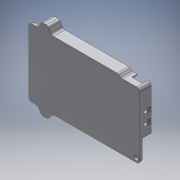
# Autodesk Inventor part: Case_superior_nuevo
Saved by Autodesk Inventor 2019 (Build 230136000, 136)
## iProperties
Created: 2018-11-21
Part Number: Case_superior_nuevo
Material: Steel, Mild, Welded
Document SubType Name: Modeling
Designer: cadcae
Density: 7.85 g/cm^3
Appearance: Smooth - White
Author: cadcae
Autodesk Inventor part; units mm, degrees
ref_plane "YZ Plane" through (0, 0, 0) normal (1, 0, 0) x (0, 1, 0)
ref_plane "XZ Plane" through (0, 0, 0) normal (0, 1, 0) x (-1, 0, 0)
ref_plane "XY Plane" through (0, 0, 0) normal (0, 0, 1) x (1, 0, 0)
sketch "Sketch1" plane through (0, 0, 0) normal (0, 0, 1) x (1, 0, 0)
  line L0 (26.8957, -31.2712) -> (26.8957, -23.2912) projected
  line L1 (26.8957, -23.2912) -> (21.7957, -23.2912) projected
  arc A0 (21.7957, -23.2912) -> (19.7957, -25.2912) centre (21.7957, -25.2912) ccw projected
  line L2 (19.7957, -25.2912) -> (19.7957, -28.2712) projected
  line L3 (19.7957, -28.2712) -> (1.7957, -28.2712) projected
  line L4 (1.7957, -28.2712) -> (1.7957, -25.2912) projected
  arc A1 (1.7957, -25.2912) -> (-0.2043, -23.2912) centre (-0.2043, -25.2912) ccw projected
  line L5 (-0.2043, -23.2912) -> (-1.3443, -23.2912) projected
  arc A2 (-1.3443, -23.2912) -> (-3.3443, -25.2912) centre (-1.3443, -25.2912) ccw projected
  line L6 (-3.3443, -25.2912) -> (-3.3443, -29.2712) projected
  line L7 (-3.3443, -29.2712) -> (-48.3643, -29.2712) projected
  line L8 (-48.3643, -29.2712) -> (-48.3643, -13.3852) projected
  line L9 (-48.3643, -13.3852) -> (-51.3643, -13.3852) projected
  line L10 (-51.3643, -13.3852) -> (-51.3643, -28.2712) projected
  arc A3 (-51.3643, -28.2712) -> (-48.3643, -31.2712) centre (-48.3643, -28.2712) ccw projected
  line L11 (-48.3643, -31.2712) -> (-44.5605, -31.2712) projected
  arc A4 (-41.9624, -32.7712) -> (-44.5605, -31.2712) centre (-44.5605, -34.2712) ccw projected
  line L12 (-40.2304, -35.7712) -> (-41.9624, -32.7712) projected
  arc A5 (-40.2304, -35.7712) -> (-37.6323, -37.2712) centre (-37.6323, -34.2712) ccw projected
  line L13 (-35.0964, -37.2712) -> (-37.6323, -37.2712) projected
  arc A6 (-35.0964, -37.2712) -> (-32.4983, -35.7712) centre (-35.0964, -34.2712) ccw projected
  line L14 (-30.7663, -32.7712) -> (-32.4983, -35.7712) projected
  arc A7 (-28.1682, -31.2712) -> (-30.7663, -32.7712) centre (-28.1682, -34.2712) ccw projected
  line L15 (-28.1682, -31.2712) -> (26.8957, -31.2712) projected
  line L16 (-45.3643, 31.7788) -> (-45.3643, 28.7788) projected
  line L17 (-45.3643, 28.7788) -> (22.8137, 28.7788) projected
  line L18 (22.8137, 28.7788) -> (24.1137, 30.2788) projected
  line L19 (24.1137, 30.2788) -> (28.1137, 30.2788) projected
  line L20 (28.1137, 30.2788) -> (29.4137, 28.7788) projected
  line L21 (29.4137, 28.7788) -> (39.3157, 28.7788) projected
  line L22 (39.3157, 28.7788) -> (39.3157, 29.7218) projected
  line L23 (39.3157, 29.7218) -> (35.9475, 29.7218) projected
  arc A8 (34.4475, 30.1238) -> (35.9475, 29.7218) centre (35.9475, 32.7218) ccw projected
  line L24 (34.4475, 30.1238) -> (32.277, 31.3769) projected
  arc A9 (32.277, 31.3769) -> (30.777, 31.7788) centre (30.777, 28.7788) ccw projected
  line L25 (30.777, 31.7788) -> (-28.1682, 31.7788) projected
  arc A10 (-30.7663, 33.2788) -> (-28.1682, 31.7788) centre (-28.1682, 34.7788) ccw projected
  line L26 (-32.4983, 36.2788) -> (-30.7663, 33.2788) projected
  arc A11 (-32.4983, 36.2788) -> (-35.0964, 37.7788) centre (-35.0964, 34.7788) ccw projected
  line L27 (-37.6323, 37.7788) -> (-35.0964, 37.7788) projected
  arc A12 (-37.6323, 37.7788) -> (-40.2304, 36.2788) centre (-37.6323, 34.7788) ccw projected
  line L28 (-41.9624, 33.2788) -> (-40.2304, 36.2788) projected
  arc A13 (-44.5605, 31.7788) -> (-41.9624, 33.2788) centre (-44.5605, 34.7788) ccw projected
  line L29 (-44.5605, 31.7788) -> (-45.3643, 31.7788) projected
  line L30 (48.8957, -11.2712) -> (51.8957, -11.2712) projected
  line L31 (51.8957, -11.2712) -> (51.8957, 26.7218) projected
  arc A14 (51.8957, 26.7218) -> (48.8957, 29.7218) centre (48.8957, 26.7218) ccw projected
  line L32 (48.8957, 29.7218) -> (48.3157, 29.7218) projected
  line L33 (48.3157, 29.7218) -> (48.3157, 28.7788) projected
  line L34 (48.3157, 28.7788) -> (48.8957, 28.7788) projected
  line L35 (48.8957, 28.7788) -> (48.8957, -11.2712) projected
  line L36 (-48.3643, 6.9348) -> (-51.3643, 6.9348) projected
  line L37 (-51.3643, 6.9348) -> (-51.3643, -4.2412) projected
  line L38 (-51.3643, -4.2412) -> (-48.3643, -4.2412) projected
  line L39 (-48.3643, -4.2412) -> (-48.3643, 6.9348) projected
  line L40 (-48.3643, -13.3852) -> (-51.3643, -13.3852)
  line L41 (-51.3643, -4.2412) -> (-48.3643, -4.2412)
  line L42 (-48.3643, 6.9348) -> (-51.3643, 6.9348)
  line L43 (-51.3643, 6.9348) -> (-51.3643, 16.0788)
  line L44 (-51.3643, 16.0788) -> (-48.3643, 16.0788)
  line L45 (-48.3643, 16.0788) -> (-48.3643, 6.9348)
  line L46 (-48.3643, 18.7788) -> (-51.3643, 18.7788) projected
  line L47 (-51.3643, 18.7788) -> (-51.3643, 16.0788) projected
  line L48 (-51.3643, 16.0788) -> (-48.3643, 16.0788) projected
  line L49 (-48.3643, 16.0788) -> (-48.3643, 18.7788) projected
  line L50 (-48.3643, -13.3852) -> (-51.3643, -13.3852)
  line L51 (-51.3643, -13.3852) -> (-51.3643, -4.2412)
  line L52 (-51.3643, -4.2412) -> (-48.3643, -4.2412)
  line L53 (-48.3643, -4.2412) -> (-48.3643, -13.3852)
  line L54 (48.3157, 29.7218) -> (48.3157, 28.7788) projected
  line L55 (39.3157, 29.7218) -> (48.3157, 29.7218) projected
  line L56 (39.3157, 28.7788) -> (39.3157, 29.7218) projected
  line L57 (48.3157, 28.7788) -> (39.3157, 28.7788) projected
  point P0 (0, 0)
  constraints: 20 end point, 6 point on line, 5 parallel, 3 horizontal, 2 perpendicular
extrude "Extrusion1" add sketch "Sketch1" along normal blind 8.6
sketch "Sketch2" plane through (0, 0, 8.6) normal (0, 0, 1) x (1, 0, 0)
  line L0 (26.8957, -31.2712) -> (26.8957, -23.2912) projected
  line L1 (26.8957, -23.2912) -> (21.7957, -23.2912) projected
  arc A0 (21.7957, -23.2912) -> (19.7957, -25.2912) centre (21.7957, -25.2912) ccw projected
  line L2 (19.7957, -25.2912) -> (19.7957, -28.2712) projected
  line L3 (19.7957, -28.2712) -> (1.7957, -28.2712) projected
  line L4 (1.7957, -28.2712) -> (1.7957, -25.2912) projected
  arc A1 (1.7957, -25.2912) -> (-0.2043, -23.2912) centre (-0.2043, -25.2912) ccw projected
  line L5 (-0.2043, -23.2912) -> (-1.3443, -23.2912) projected
  arc A2 (-1.3443, -23.2912) -> (-3.3443, -25.2912) centre (-1.3443, -25.2912) ccw projected
  line L6 (-3.3443, -25.2912) -> (-3.3443, -29.2712) projected
  line L7 (-3.3443, -29.2712) -> (-48.3643, -29.2712) projected
  line L8 (-48.3643, -29.2712) -> (-48.3643, 18.7788) projected
  line L9 (-51.3643, 18.7788) -> (-51.3643, -28.2712) projected
  arc A3 (-51.3643, -28.2712) -> (-48.3643, -31.2712) centre (-48.3643, -28.2712) ccw projected
  line L10 (-48.3643, -31.2712) -> (-44.5605, -31.2712) projected
  arc A4 (-41.9624, -32.7712) -> (-44.5605, -31.2712) centre (-44.5605, -34.2712) ccw projected
  line L11 (-41.9624, -32.7712) -> (-40.2304, -35.7712) projected
  arc A5 (-40.2304, -35.7712) -> (-37.6323, -37.2712) centre (-37.6323, -34.2712) ccw projected
  line L12 (-37.6323, -37.2712) -> (-35.0964, -37.2712) projected
  arc A6 (-35.0964, -37.2712) -> (-32.4983, -35.7712) centre (-35.0964, -34.2712) ccw projected
  line L13 (-32.4983, -35.7712) -> (-30.7663, -32.7712) projected
  arc A7 (-28.1682, -31.2712) -> (-30.7663, -32.7712) centre (-28.1682, -34.2712) ccw projected
  line L14 (-28.1682, -31.2712) -> (26.8957, -31.2712) projected
  line L15 (-48.3643, 18.7788) -> (-51.3643, 18.7788) projected
  line L16 (-48.3643, 28.7788) -> (-45.3643, 28.7788) projected
  line L17 (-45.3643, 28.7788) -> (-45.3643, 31.7788) projected
  line L18 (-45.3643, 31.7788) -> (-48.3643, 31.7788) projected
  arc A8 (-48.3643, 31.7788) -> (-51.3643, 28.7788) centre (-48.3643, 28.7788) ccw projected
  line L19 (-51.3643, 28.7788) -> (-51.3643, 18.7788) projected
  line L20 (-51.3643, 18.7788) -> (-48.3643, 18.7788) projected
  line L21 (-48.3643, 18.7788) -> (-48.3643, 28.7788) projected
  line L22 (29.4137, 28.7788) -> (48.8957, 28.7788) projected
  line L23 (48.8957, 28.7788) -> (48.8957, -11.2712) projected
  line L24 (48.8957, -11.2712) -> (51.8957, -11.2712) projected
  line L25 (51.8957, -11.2712) -> (51.8957, 26.7218) projected
  arc A9 (51.8957, 26.7218) -> (48.8957, 29.7218) centre (48.8957, 26.7218) ccw projected
  line L26 (48.8957, 29.7218) -> (35.9475, 29.7218) projected
  arc A10 (34.4475, 30.1238) -> (35.9475, 29.7218) centre (35.9475, 32.7218) ccw projected
  line L27 (34.4475, 30.1238) -> (32.277, 31.3769) projected
  arc A11 (32.277, 31.3769) -> (30.777, 31.7788) centre (30.777, 28.7788) ccw projected
  line L28 (30.777, 31.7788) -> (-28.1682, 31.7788) projected
  arc A12 (-30.7663, 33.2788) -> (-28.1682, 31.7788) centre (-28.1682, 34.7788) ccw projected
  line L29 (-30.7663, 33.2788) -> (-32.4983, 36.2788) projected
  arc A13 (-32.4983, 36.2788) -> (-35.0964, 37.7788) centre (-35.0964, 34.7788) ccw projected
  line L30 (-35.0964, 37.7788) -> (-37.6323, 37.7788) projected
  arc A14 (-37.6323, 37.7788) -> (-40.2304, 36.2788) centre (-37.6323, 34.7788) ccw projected
  line L31 (-40.2304, 36.2788) -> (-41.9624, 33.2788) projected
  arc A15 (-44.5605, 31.7788) -> (-41.9624, 33.2788) centre (-44.5605, 34.7788) ccw projected
  line L32 (-44.5605, 31.7788) -> (-45.3643, 31.7788) projected
  line L33 (-45.3643, 31.7788) -> (-45.3643, 28.7788) projected
  line L34 (-45.3643, 28.7788) -> (22.8137, 28.7788) projected
  line L35 (22.8137, 28.7788) -> (24.1137, 30.2788) projected
  line L36 (24.1137, 30.2788) -> (28.1137, 30.2788) projected
  line L37 (28.1137, 30.2788) -> (29.4137, 28.7788) projected
  arc A16 (48.8957, -31.2712) -> (51.8957, -28.2712) centre (48.8957, -28.2712) ccw projected
  line L38 (51.8957, -28.2712) -> (51.8957, -11.2712) projected
  line L39 (51.8957, -11.2712) -> (48.8957, -11.2712) projected
  line L40 (48.8957, -11.2712) -> (48.8957, -23.2912) projected
  line L41 (48.8957, -23.2912) -> (26.8957, -23.2912) projected
  line L42 (26.8957, -23.2912) -> (26.8957, -31.2712) projected
  line L43 (26.8957, -31.2712) -> (48.8957, -31.2712) projected
  point P0 (0, 0)
extrude "Extrusion2" add sketch "Sketch2" along normal blind 2 contours L14 A7 L13 A6 L12 A5 L11 A4 L10 A3 L9 L15 L8 L7 L6 A2 L5 A1 L4 L3 L2 A0 L1 L0 | L0 L41 L40 L24 L38 A16 L43 | L23 L22 L37 L36 L35 L34 L17 L32 A15 L31 A14 L30 A13 L29 A12 L28 A11 L27 A10 L26 A9 L25 L24 | L16 L21 L15 L19 A8 L18 L17
sketch "Sketch3" plane through (-48.3643, -29.2712, 0) normal (1, 0, 0) x (0, 0, -1)
  line L0 (0, 48.05) -> (0, 1) projected
  line L1 (0, 1) -> (-10.6, 1) projected
  line L2 (-10.6, 58.05) -> (-10.6, 1) projected
  line L3 (-8.6, 58.05) -> (-10.6, 58.05) projected
  line L4 (-8.6, 58.05) -> (-8.6, 48.05) projected
  line L5 (0, 48.05) -> (-8.6, 48.05) projected
  line L6 (-8.6, 61.05) -> (-8.6, 58.05) projected
  line L7 (-8.6, 58.05) -> (-10.6, 58.05) projected
  line L8 (-10.6, 61.05) -> (-10.6, 58.05) projected
  line L9 (-8.6, 61.05) -> (-10.6, 61.05) projected
  line L10 (0, 1) -> (0, -2) projected
  line L11 (0, -2) -> (-10.6, -2) projected
  line L12 (-10.6, 1) -> (-10.6, -2) projected
  line L13 (0, 1) -> (-10.6, 1) projected
  line L14 (-10.6, -2) -> (-8.6, -2)
  line L15 (-8.6, -2) -> (-8.6, 61.05)
  line L16 (-8.6, 61.05) -> (-10.6, 61.05)
  line L17 (-10.6, 61.05) -> (-10.6, -2)
  point P0 (0, 29.2712)
  dimension "d4" = 2
  constraints: 8 end point, 2 parallel, 1 horizontal, 1 perpendicular
  measures "d4" distance of L15.end L8.start
extrude "Extrusion3" add sketch "Sketch3" along normal up to surface (97.26 mm away) contours L15 L1 L2 L3 L4 | L15 L11 L12 L1
extrude "Extrusion4" add sketch "Sketch3" along normal up to surface (77.778 mm away) contours L3 L8 L9 L6
sketch "Sketch4" plane through (-51.3643, -28.2712, 0) normal (-1, 0, 0) x (0, 0, 1)
  circle A0 centre (0, 39.778) radius 4.572
  circle A1 centre (0, 19.458) radius 4.572
  line L0 (0, 47.05) -> (0, 0) projected
  line L1 (0, 0) -> (10.6, 0) projected
  line L2 (10.6, 57.05) -> (10.6, 0) projected
  line L3 (8.6, 57.05) -> (10.6, 57.05) projected
  line L4 (8.6, 57.05) -> (8.6, 47.05) projected
  line L5 (0, 47.05) -> (8.6, 47.05) projected
  line L6 (0, 47.05) -> (0, 0) projected
  point P0 (0, 28.2712)
  dimension "d9" = 7.272
  dimension "d10" = 20.32
  dimension "d13" = 9.144
  constraints: 2 centre point, 1 equal radius, 1 point on line, 1 vertical alignment
  measures "d9" distance from line of A0.centre L5
  measures "d10" distance of A1.centre A0.centre
  measures "d13" diameter of A0
extrude "Extrusion5" cut sketch "Sketch4" against normal blind 10 contours A0 L0 | L0 A0 | L0 A1 | A1 L0
sketch "Sketch5" plane through (35.9475, 29.7218, 0) normal (0, 1, 0) x (1, 0, 0)
  line L0 (12.3682, -4.5974) -> (3.3682, -4.5974)
  line L1 (3.3682, -4.5974) -> (3.3682, 0)
  line L2 (3.3682, 0) -> (12.3682, 0)
  line L3 (12.3682, 0) -> (12.3682, -4.5974)
  line L4 (12.9482, 0) -> (0, 0) projected
  line L5 (0, 0) -> (0, -10.6) projected
  line L6 (12.9482, -10.6) -> (0, -10.6) projected
  line L7 (12.9482, 0) -> (12.9482, -10.6) projected
  line L8 (15.9482, 0) -> (12.9482, 0) projected
  line L9 (12.9482, 0) -> (12.9482, -10.6) projected
  line L10 (15.9482, -10.6) -> (12.9482, -10.6) projected
  line L11 (15.9482, 0) -> (15.9482, -10.6) projected
  line L12 (12.9482, 0) -> (0, 0) projected
  point P0 (-35.9475, 0)
  dimension "d14" = 4.5974
  dimension "d15" = 3.58
  dimension "d16" = 9
  constraints: 8 end point, 2 parallel, 1 horizontal, 1 perpendicular, 1 point on line
  measures "d14" distance between parallel lines of L4 L0
  measures "d15" distance between parallel lines of L3 L11
  measures "d16" distance of L1.end L2.end
extrude "Extrusion6" cut sketch "Sketch5" against normal up to next contours L0 L1 L2 L3
sketch "Sketch6" plane through (51.8957, -11.2712, 0) normal (1, 0, 0) x (0, 0, -1)
  line L0 (0, 0) -> (0, 37.993) projected
  line L1 (0, 37.993) -> (-10.6, 37.993) projected
  line L2 (-10.6, -17) -> (-10.6, 37.993) projected
  line L3 (-8.6, -17) -> (-10.6, -17) projected
  line L4 (-8.6, -17) -> (-8.6, 0) projected
  line L5 (0, 0) -> (-8.6, 0) projected
  circle A0 centre (-5.3, 10) radius 1.5
  circle A1 centre (-5.3, 20) radius 1.5
  point P0 (0, 11.2712)
  point P1 (-5.3, 37.993)
  dimension "d19" = 10
  dimension "d20" = 10
  dimension "d21" = 3
  constraints: 2 centre point, 2 vertical alignment, 1 equal radius, 1 midpoint
  measures "d19" distance from line of L5 A0.centre
  measures "d20" distance of A1.centre A0.centre
  measures "d21" diameter of A0
extrude "Extrusion7" cut sketch "Sketch6" against normal up to next contours A0 | A1
sketch "Sketch7" plane through (51.8957, -11.2712, 0) normal (1, 0, 0) x (0, 0, -1)
  line L0 (-3.2, 7.3511) -> (-3.2, 12.6489) construction
  line L1 (-3.2, 12.6489) -> (-0.5947, 12.6489) construction
  line L2 (-0.5947, 12.6489) -> (-0.5947, 7.3511) construction
  line L3 (-0.5947, 7.3511) -> (-3.2, 7.3511) construction
  line L4 (-3.2, 17.6246) -> (-3.2, 22.3754) construction
  line L5 (-3.2, 22.3754) -> (-0.5987, 22.3754) construction
  line L6 (-0.5987, 22.3754) -> (-0.5987, 17.6246) construction
  line L7 (-0.5987, 17.6246) -> (-3.2, 17.6246) construction
  circle A0 centre (-5.3, 10) radius 1.5 projected
  circle A1 centre (-5.3, 20) radius 1.5 projected
  line L8 (0, 0) -> (0, 37.993) projected
  line L9 (0, 37.993) -> (-10.6, 37.993) projected
  line L10 (-10.6, -17) -> (-10.6, 37.993) projected
  line L11 (-8.6, -17) -> (-10.6, -17) projected
  line L12 (-8.6, -17) -> (-8.6, 0) projected
  line L13 (0, 0) -> (-8.6, 0) projected
  spline S0 degree 2 poles (-1.8973, 9.8855) (-1.2895, 9.8855) (-0.5947, 9.2372) (-0.5947, 8.674) knots 0 0 0 1 2 2 2
  spline S1 degree 2 poles (-0.5947, 8.674) (-0.5947, 8.1088) (-1.2977, 7.4645) (-1.8973, 7.4645) knots 0 0 0 1 2 2 2
  spline S2 degree 2 poles (-1.8973, 7.4645) (-2.499, 7.4645) (-3.2, 8.1088) (-3.2, 8.674) knots 0 0 0 1 2 2 2
  spline S3 degree 2 poles (-3.2, 8.674) (-3.2, 9.2372) (-2.5031, 9.8855) (-1.8973, 9.8855) knots 0 0 0 1 2 2 2
  spline S4 degree 2 poles (-1.8973, 9.2372) (-2.1222, 9.2372) (-2.4362, 9.1461) (-2.5355, 9.0671) knots 0 0 0 1 2 2 2
  spline S5 degree 2 poles (-2.5355, 9.0671) (-2.6388, 8.988) (-2.728, 8.7855) (-2.728, 8.6761) knots 0 0 0 1 2 2 2
  spline S6 degree 2 poles (-2.728, 8.6761) (-2.728, 8.5606) (-2.6449, 8.3722) (-2.5395, 8.285) knots 0 0 0 1 2 2 2
  spline S7 degree 2 poles (-2.5395, 8.285) (-2.4423, 8.2081) (-2.1202, 8.1128) (-1.8973, 8.1128) knots 0 0 0 1 2 2 2
  spline S8 degree 2 poles (-1.8973, 8.1128) (-1.6664, 8.1128) (-1.3625, 8.204) (-1.2592, 8.283) knots 0 0 0 1 2 2 2
  spline S9 degree 2 poles (-1.2592, 8.283) (-1.1558, 8.362) (-1.0667, 8.5667) (-1.0667, 8.6761) knots 0 0 0 1 2 2 2
  spline S10 degree 2 poles (-1.0667, 8.6761) (-1.0667, 8.7875) (-1.1619, 8.9941) (-1.2632, 9.0691) knots 0 0 0 1 2 2 2
  spline S11 degree 2 poles (-1.2632, 9.0691) (-1.3726, 9.1501) (-1.6623, 9.2372) (-1.8973, 9.2372) knots 0 0 0 1 2 2 2
  line L14 (-0.6473, 12.3997) -> (-0.6473, 11.796)
  line L15 (-0.6473, 11.796) -> (-2.3896, 10.8316)
  line L16 (-2.3896, 10.8316) -> (-0.6473, 10.8316)
  line L17 (-0.6473, 10.8316) -> (-0.6473, 10.2583)
  line L18 (-0.6473, 10.2583) -> (-3.1473, 10.2583)
  line L19 (-3.1473, 10.2583) -> (-3.1473, 11.0282)
  line L20 (-3.1473, 11.0282) -> (-1.715, 11.8264)
  line L21 (-1.715, 11.8264) -> (-3.1473, 11.8264)
  line L22 (-3.1473, 11.8264) -> (-3.1473, 12.3997)
  line L23 (-3.1473, 12.3997) -> (-0.6473, 12.3997)
  line L24 (-0.6514, 19.7154) -> (-0.6514, 17.8778)
  line L25 (-0.6514, 17.8778) -> (-1.0586, 17.8778)
  spline S12 degree 2 poles (-1.0586, 17.8778) (-1.245, 18.1108) (-1.5732, 18.4836) (-1.7211, 18.6234) knots 0 0 0 1 2 2 2
  spline S13 degree 2 poles (-1.7211, 18.6234) (-1.9135, 18.8077) (-2.2073, 18.9718) (-2.3613, 18.9718) knots 0 0 0 1 2 2 2
  spline S14 degree 2 poles (-2.3613, 18.9718) (-2.5355, 18.9718) (-2.7219, 18.7632) (-2.7219, 18.5768) knots 0 0 0 1 2 2 2
  spline S15 degree 2 poles (-2.7219, 18.5768) (-2.7219, 18.4816) (-2.6753, 18.3114) (-2.6388, 18.2243) knots 0 0 0 1 2 2 2
  spline S16 degree 2 poles (-2.6388, 18.2243) (-2.6003, 18.1392) (-2.5193, 18.0176) (-2.499, 17.9872) knots 0 0 0 1 2 2 2
  line L26 (-2.499, 17.9872) -> (-2.499, 17.9386)
  line L27 (-2.499, 17.9386) -> (-3.044, 17.9386)
  spline S17 degree 2 poles (-3.044, 17.9386) (-3.0947, 18.044) (-3.2, 18.4937) (-3.2, 18.7024) knots 0 0 0 1 2 2 2
  spline S18 degree 2 poles (-3.2, 18.7024) (-3.2, 19.1481) (-2.8029, 19.606) (-2.4443, 19.606) knots 0 0 0 1 2 2 2
  spline S19 degree 2 poles (-2.4443, 19.606) (-2.2235, 19.606) (-1.7981, 19.3973) (-1.5549, 19.1562) knots 0 0 0 1 2 2 2
  spline S20 degree 2 poles (-1.5549, 19.1562) (-1.405, 19.0043) (-1.172, 18.7186) (-1.1234, 18.6558) knots 0 0 0 1 2 2 2
  line L28 (-1.1234, 18.6558) -> (-1.1234, 19.7154)
  line L29 (-1.1234, 19.7154) -> (-0.6514, 19.7154)
  spline S21 degree 2 poles (-0.7932, 22.1607) (-0.7263, 21.9966) (-0.5987, 21.4718) (-0.5987, 21.2166) knots 0 0 0 1 2 2 2
  spline S22 degree 2 poles (-0.5987, 21.2166) (-0.5987, 20.627) (-1.2794, 19.9281) (-1.9034, 19.9281) knots 0 0 0 1 2 2 2
  spline S23 degree 2 poles (-1.9034, 19.9281) (-2.4909, 19.9281) (-3.2, 20.627) (-3.2, 21.2348) knots 0 0 0 1 2 2 2
  spline S24 degree 2 poles (-3.2, 21.2348) (-3.2, 21.5488) (-3.0805, 21.9419) (-2.9792, 22.1505) knots 0 0 0 1 2 2 2
  line L30 (-2.9792, 22.1505) -> (-2.3917, 22.1505)
  line L31 (-2.3917, 22.1505) -> (-2.3917, 22.0938)
  spline S25 degree 2 poles (-2.3917, 22.0938) (-2.4261, 22.0492) (-2.5578, 21.8791) (-2.6024, 21.798) knots 0 0 0 1 2 2 2
  spline S26 degree 2 poles (-2.6024, 21.798) (-2.6571, 21.7048) (-2.734, 21.4577) (-2.734, 21.3199) knots 0 0 0 1 2 2 2
  spline S27 degree 2 poles (-2.734, 21.3199) (-2.734, 21.1598) (-2.6327, 20.8944) (-2.5294, 20.7911) knots 0 0 0 1 2 2 2
  spline S28 degree 2 poles (-2.5294, 20.7911) (-2.4281, 20.6919) (-2.1182, 20.5764) (-1.9135, 20.5764) knots 0 0 0 1 2 2 2
  spline S29 degree 2 poles (-1.9135, 20.5764) (-1.4759, 20.5764) (-1.0586, 21.016) (-1.0586, 21.3949) knots 0 0 0 1 2 2 2
  spline S30 degree 2 poles (-1.0586, 21.3949) (-1.0586, 21.4293) (-1.0626, 21.5184) (-1.0647, 21.5529) knots 0 0 0 1 2 2 2
  line L32 (-1.0647, 21.5529) -> (-1.557, 21.5529)
  line L33 (-1.557, 21.5529) -> (-1.557, 21.0687)
  line L34 (-1.557, 21.0687) -> (-2.025, 21.0687)
  line L35 (-2.025, 21.0687) -> (-2.025, 22.1607)
  line L36 (-2.025, 22.1607) -> (-0.7932, 22.1607)
  point P0 (0, 11.2712)
  point P1 (-3.2, 10)
  point P2 (-3.2, 20)
  dimension "d24" = 2.1
  constraints: 2 horizontal alignment, 2 midpoint, 1 vertical alignment, 4 other
  measures "d24" distance of point (-3.2, 20) A1.centre
extrude "Extrusion8" cut sketch "Sketch7" against normal blind 0.25 contours S0 S1 S2 S3 | L14 L15 L16 L17 L18 L19 L20 L21 L22 L23 | L24 L25 S12 S13 S14 S15 S16 L26 L27 S17 S18 S19 S20 L28 L29 | S21 S22 S23 S24 L30 L31 S25 S26 S27 S28 S29 S30 L32 L33 L34 L35 L36
sketch "Sketch8" plane through (0, 0, 0) normal (0, 0, -1) x (-1, 0, 0)
  arc A0 (41.9624, 33.2788) -> (44.5605, 31.7788) centre (44.5605, 34.7788) ccw
  line L0 (37.6323, 37.7788) -> (35.0964, 37.7788)
  line L1 (32.4983, 36.2788) -> (30.7663, 33.2788)
  line L2 (41.9624, 33.2788) -> (40.2304, 36.2788)
  circle A1 centre (36.3643, 34.7788) radius 1.8
  line L3 (35.0964, 37.7788) -> (37.6323, 37.7788) projected
  line L4 (35.0964, -37.2712) -> (37.6323, -37.2712)
  circle A2 centre (36.3643, -34.2712) radius 1.8
  point P0 (0, 0)
  point P1 (36.3643, 37.7788)
  point P2 (36.3643, 37.7788)
  point P3 (36.3643, -37.2712)
  dimension "d27" = 3.6
  dimension "d28" = 3
  dimension "d29" = 3.6
  dimension "d30" = 3
  constraints: 8 end point, 3 centre point, 3 midpoint, 2 horizontal, 2 point on circle, 2 vertical alignment, 13 other
  measures "d27" diameter of A1
  measures "d28" distance from line of A1.centre L0
  measures "d29" diameter of A2
  measures "d30" distance from line of L4 A2.centre
extrude "Extrusion9" cut sketch "Sketch8" against normal blind 4
sketch "Sketch10" plane through (0, 0, 10.6) normal (0, 0, 1) x (1, 0, 0)
  point P0 (48.2957, -27.6712)
hole "Hole1" at (48.2957, -27.6712, 10.6) direction (0, 0, -1) diameter 2.4 depth 2 countersink diameter 4.4 countersink angle 90
sketch "Sketch11" plane through (35.9475, 29.7218, 10.6) normal (0, 1, 0) x (1, 0, 0)
  line L0 (3.3682, 6.0026) -> (3.3682, 10.6) projected
  line L1 (3.3682, 10.6) -> (0, 10.6) projected
  line L2 (0, 10.6) -> (0, 0) projected
  line L3 (12.9482, 0) -> (0, 0) projected
  line L4 (12.9482, 10.6) -> (12.9482, 0) projected
  line L5 (12.9482, 10.6) -> (12.3682, 10.6) projected
  line L6 (12.3682, 10.6) -> (12.3682, 6.0026) projected
  line L7 (12.3682, 6.0026) -> (3.3682, 6.0026) projected
  line L8 (12.9482, 10.6) -> (12.9482, 5.5026)
  line L9 (12.9482, 5.5026) -> (2.8682, 5.5026)
  line L10 (2.8682, 5.5026) -> (2.8682, 10.6)
  line L11 (3.3682, 10.6) -> (0, 10.6) projected
  point P0 (-35.9475, 10.6)
  dimension "d40" = 0.5
  dimension "d41" = 0.5
  constraints: 6 end point, 2 perpendicular, 1 point on line, 1 vertical
  measures "d40" distance between parallel lines of L9 L7
  measures "d41" distance between parallel lines of L0 L10
extrude "Extrusion10" cut sketch "Sketch11" against normal up to surface (0.943 mm away) contours L7 L6 L5 L4 L9 L10 L1 L0
sketch "Sketch12" plane through (0, 0, 0) normal (0, 0, -1) x (-1, 0, 0)
  circle A0 centre (36.3643, -34.2712) radius 1.8 projected
  line L0 (51.3643, -13.3852) -> (48.3643, -13.3852) projected
  line L1 (48.3643, -29.2712) -> (48.3643, -13.3852) projected
  line L2 (3.3443, -29.2712) -> (48.3643, -29.2712) projected
  line L3 (3.3443, -25.2912) -> (3.3443, -29.2712) projected
  arc A1 (3.3443, -25.2912) -> (1.3443, -23.2912) centre (1.3443, -25.2912) ccw projected
  line L4 (0.2043, -23.2912) -> (1.3443, -23.2912) projected
  arc A2 (0.2043, -23.2912) -> (-1.7957, -25.2912) centre (0.2043, -25.2912) ccw projected
  line L5 (-1.7957, -28.2712) -> (-1.7957, -25.2912) projected
  line L6 (-19.7957, -28.2712) -> (-1.7957, -28.2712) projected
  line L7 (-19.7957, -25.2912) -> (-19.7957, -28.2712) projected
  arc A3 (-19.7957, -25.2912) -> (-21.7957, -23.2912) centre (-21.7957, -25.2912) ccw projected
  line L8 (-26.8957, -23.2912) -> (-21.7957, -23.2912) projected
  line L9 (-26.8957, -31.2712) -> (-26.8957, -23.2912) projected
  line L10 (28.1682, -31.2712) -> (-26.8957, -31.2712) projected
  arc A4 (30.7663, -32.7712) -> (28.1682, -31.2712) centre (28.1682, -34.2712) ccw projected
  line L11 (32.4983, -35.7712) -> (30.7663, -32.7712) projected
  arc A5 (32.4983, -35.7712) -> (35.0964, -37.2712) centre (35.0964, -34.2712) ccw projected
  line L12 (37.6323, -37.2712) -> (35.0964, -37.2712) projected
  arc A6 (37.6323, -37.2712) -> (40.2304, -35.7712) centre (37.6323, -34.2712) ccw projected
  line L13 (41.9624, -32.7712) -> (40.2304, -35.7712) projected
  arc A7 (44.5605, -31.2712) -> (41.9624, -32.7712) centre (44.5605, -34.2712) ccw projected
  line L14 (48.3643, -31.2712) -> (44.5605, -31.2712) projected
  arc A8 (48.3643, -31.2712) -> (51.3643, -28.2712) centre (48.3643, -28.2712) ccw projected
  line L15 (51.3643, -13.3852) -> (51.3643, -28.2712) projected
  line L16 (-1.7957, -28.2712) -> (3.3443, -28.2712)
  point P0 (0, 0)
  constraints: 2 end point, 1 perpendicular, 1 point on line
extrude "Extrusion11" cut sketch "Sketch12" against normal up to surface (8.6 mm away) contours L16 L5 A2 L4 A1 L3
fillet "Fillet1" radius 2 1 edges at (-3.3443, -28.2712, 4.3)
body "Solid1"
